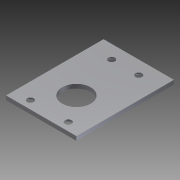
# Autodesk Inventor part: 13_1087_021
Saved by Autodesk Inventor 2014 (Build 180170000, 170)
## iProperties
Created: 2013-09-10
Part Number: 13_1087_021
Material: Allgemein
Document SubType Name: Modeling
Designer: vogel
Density: 1 g/cm^3
Appearance: Vorgabe
Author: vogel
Autodesk Inventor part; units mm, degrees
ref_plane "YZ Plane" through (0, 0, 0) normal (1, 0, 0) x (0, 1, 0)
ref_plane "XZ Plane" through (0, 0, 0) normal (0, 1, 0) x (-1, 0, 0)
ref_plane "XY Plane" through (0, 0, 0) normal (0, 0, 1) x (1, 0, 0)
sketch "Skizze1" plane through (0, 0, 0) normal (0, 0, 1) x (1, 0, 0)
  line L0 (-5.2, 0) -> (31.2, 0) projected
  line L1 (0, -7.2) -> (0, 43.2) projected
  line L2 (0, 0) -> (26, 0)
  line L3 (26, 0) -> (26, 36)
  line L4 (26, 36) -> (0, 36)
  line L5 (0, 36) -> (0, 0)
  dimension "d0" = 36
  dimension "d1" = 26
  constraints: 8 end point, 2 parallel, 1 horizontal, 1 perpendicular
  measures "d0" distance of L4.end L2.start
  measures "d1" distance of L3.end L4.end
extrude "Extrusion1" add sketch "Skizze1" along normal blind 1.5
sketch "Skizze2" plane through (0, 0, 0) normal (0, 0, -1) x (-1, 0, 0)
  circle A0 centre (-13, 13) radius 4.8 projected
  constraints: 1 coincident
hole "Bohrung1" at (13, 13, 0) direction (0, 0, 1) diameter 10.5 end through all
sketch "Skizze3" plane through (0, 0, 0) normal (0, 0, -1) x (-1, 0, 0)
  line L0 (0, 0) -> (-26, 0) projected
  line L1 (-26, 36) -> (0, 36) projected
  line L2 (-20, 31) -> (-6, 31)
  line L3 (-6, 31) -> (-6, 3)
  line L4 (-6, 3) -> (-20, 3)
  line L5 (-20, 3) -> (-20, 31)
  line L6 (-13, 36) -> (-13, 0)
  point P0 (-18, 31)
  point P1 (-8, 31)
  dimension "d11" = 28
  dimension "d12" = 14
  dimension "d20" = 3
  dimension "d21" = 10
  constraints: 10 end point, 2 coincident, 2 midpoint, 2 parallel, 2 point on line, 1 horizontal, 1 perpendicular, 1 symmetric about line, 1 other
  measures "d11" distance of L4.end L2.start
  measures "d12" distance of L3.end L4.end
  measures "d20" distance between parallel lines of L0 L4
  measures "d21" distance of point (-8, 31) point (-18, 31)
hole "Bohrung2" at (18, 31, 0) at (8, 31, 0) at (20, 3, 0) at (6, 3, 0) direction (0, 0, 1) diameter 2.4 end through all countersink diameter 4.5 countersink angle 90
